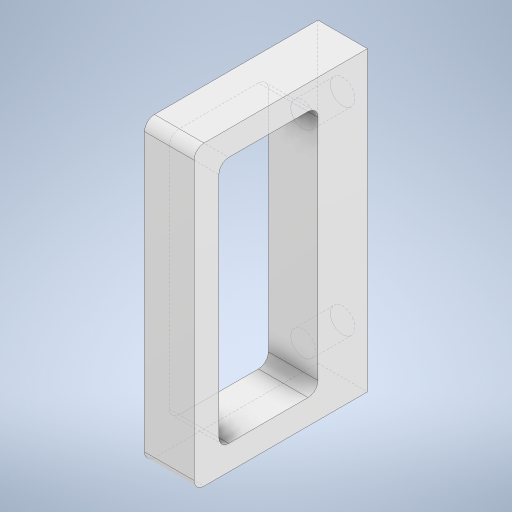
# Autodesk Inventor part: BP_BOX-handle
Saved by Autodesk Inventor 2024.3 (Build 283343000, 343)
## iProperties
Created: 2025-10-31
Part Number: BP_BOX-handle
Material: ABS プラスチック
Document SubType Name: Modeling
Designer: 佐藤智貴
Density: 1.06 g/cm^3
Appearance: 滑らか - 白
Author: 佐藤智貴
Autodesk Inventor part; units mm, degrees
ref_plane "YZ Plane" through (0, 0, 0) normal (1, 0, 0) x (0, 1, 0)
ref_plane "XZ Plane" through (0, 0, 0) normal (0, 1, 0) x (-1, 0, 0)
ref_plane "XY Plane" through (0, 0, 0) normal (0, 0, 1) x (1, 0, 0)
sketch "スケッチ1" plane through (0, 0, 0) normal (0, 0, 1) x (1, 0, 0)
  line L0 (0, 0) -> (10, 0)
  line L1 (10, 0) -> (10, 60)
  line L2 (10, 60) -> (0, 60)
  line L3 (0, 60) -> (0, 0)
  dimension "d0" = 10
  dimension "d1" = 60
  constraints: 8 end point, 2 parallel, 1 horizontal, 1 perpendicular
  measures "d0" distance of L1.end L2.end
  measures "d1" distance of L0.end L1.end
extrude "押し出し1" add sketch "スケッチ1" along normal blind 5
sketch "スケッチ3" plane through (0, 0, 5) normal (0, 0, 1) x (1, 0, 0)
  line L0 (10, 0) -> (10, 60) projected
  line L1 (10, 60) -> (0, 60) projected
  line L2 (0, 60) -> (0, 0) projected
  line L3 (0, 0) -> (10, 0) projected
  line L4 (10, 60) -> (0, 60)
  line L5 (0, 60) -> (0, 0)
  line L6 (0, 0) -> (10, 0)
  line L7 (10, 0) -> (10, 60)
  constraints: 8 end point, 2 parallel, 1 horizontal, 1 perpendicular
extrude "押し出し2" add sketch "スケッチ3" along normal blind 30
sketch "スケッチ4" plane through (10, 0, 0) normal (1, 0, 0) x (0, 0, -1)
  line L0 (0, 60) -> (-35, 60) projected
  line L1 (0, 0) -> (0, 60) projected
  line L2 (0, 0) -> (-35, 0) projected
  line L3 (-35, 60) -> (-5, 60)
  line L4 (-5, 60) -> (-5, 0)
  line L5 (-5, 0) -> (-35, 0)
  line L6 (-35, 0) -> (-35, 60)
  line L7 (-30, 55) -> (-10, 55)
  line L8 (-10, 55) -> (-10, 5)
  line L9 (-10, 5) -> (-30, 5)
  line L10 (-30, 5) -> (-30, 55)
  dimension "d37" = 5
  dimension "d38" = 5
  dimension "d39" = 20
  constraints: 16 end point, 4 parallel, 2 perpendicular, 1 horizontal, 1 point on line, 3 other
  measures "d37" distance between parallel lines of L1 L4
  measures "d38" distance between parallel lines of L0 L7
  measures "d39" distance of L7.start L7.end
extrude "押し出し3" cut sketch "スケッチ4" against normal blind 40 contours L7 L8 L9 L10
sketch "スケッチ5" plane through (0, 0, 0) normal (0, 0, -1) x (-1, 0, 0)
  line L0 (0, 60) -> (0, 0) projected
  line L1 (0, 0) -> (-10, 0) projected
  point P0 (-5, 50)
  point P1 (-5, 10)
  dimension "d23" = 40
  dimension "d24" = 5
  dimension "d25" = 5
  dimension "d26" = 10
  measures "d23" distance of point (-5, 10) point (-5, 50)
  measures "d24" distance from line of L0 point (-5, 50)
  measures "d25" distance from line of L0 point (-5, 10)
  measures "d26" distance from line of L1 point (-5, 10)
hole "穴2" at (5, 50, 0) at (5, 10, 0) direction (0, 0, 1) diameter 5 depth 8
fillet "フィレット1" radius 2 6 edges at (5, 55, 10) (5, 55, 30) (5, 5, 30) (5, 5, 10) (5, 0, 35) (5, 60, 35)
equation "\"d25\" = d24"
